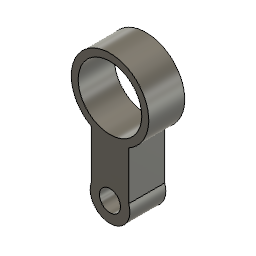
Trumpet+Clamp+4 (Autodesk Fusion 360 design; units mm, degrees)
Autodesk Fusion 360 part; units mm, degrees
note: some values were not read from the file. Chosen so that the rebuilt part matches the saved one: which face or edge a step refers to.
sketch "Sketch1" plane through (0, 0, 0) normal (0, 0, 1) x (1, 0, 0)
  circle A0 centre (0, 0) radius 2.25
  circle A1 centre (0, 0) radius 4.25
  line L0 (-4, 1.4361) -> (-4, 11.756)
  line L1 (4, 1.4361) -> (4, 11.756)
  circle A2 centre (0, 19) radius 6.775
  circle A3 centre (0, 19) radius 8.275
  line L2 (-4, 1.4361) -> (4, 1.4361) construction
  line L3 (-4, 11.756) -> (4, 11.756) construction
  line L4 (-2.7954, 26.7885) -> (-7.7596, 21.8747) construction
  line L5 (0, 0) -> (0, 19) construction
  dimension "d1" = 4.5
  dimension "d2" = 8.5
  dimension "d3" = 13.55
  dimension "d4" = 16.55
  dimension "d5" = 19
  dimension "d6" = 8
  constraint coincident A0.centre A1.centre
  constraint coincident A1 L0.start
  constraint coincident A1 L1.start
  constraint concentric A2 A3
  constraint parallel L0 L1
  constraint coincident L0.end A3
  constraint coincident L1.end A3
  constraint perpendicular L0 L2
  constraint perpendicular L0 L3
  constraint coincident A3 L4.end
  constraint coincident A3 L4.start
  constraint coincident A2.centre A3.centre
  constraint vertical L5
  measures "d1" diameter of A0
  measures "d2" diameter of A1
  measures "d3" diameter of A2
  measures "d4" diameter of A3
  measures "d5" distance of A0.centre A2.centre
  measures "d6" distance of L0 L1
extrude "Extrude1" add sketch "Sketch1" along normal blind 7.7
sketch "Sketch2" plane through (-2.8621, 2.7943, 0) normal (-0.715528, 0.698585, 0) x (0, 0, 1)
  line L0 (0, 10.5084) -> (0, 1.4361)
  line L1 (0, 1.4361) -> (7.7, 1.4361)
  line L2 (7.7, 1.4361) -> (7.7, 10.5084)
  line L3 (7.7, 10.5084) -> (0, 10.5084)
  line L4 (0, 5.9723) -> (7.7, 5.9723) construction
  line L5 (3.85, 10.5084) -> (3.85, 1.4361) construction
  circle A0 centre (3.85, 5.9723) radius 2.25
  dimension "d10" = 4.5
  constraint midpoint L0 L4.start
  constraint midpoint L2 L4.end
  constraint midpoint L3 L5.start
  constraint midpoint L1 L5.end
  constraint midpoint L5 A0.centre
  measures "d10" diameter of A0
extrude "Extrude2" [rolled back] side1offset 0 taper angle 0
sketch "Sketch3" plane through (15.0791, 0, 0) normal (1, 0, 0) x (0, 0, -1)
  line L0 (0, 19.0835) -> (0, 31.0835)
  line L1 (0, 31.0835) -> (-7.7, 31.0835)
  line L2 (-7.7, 31.0835) -> (-7.7, 19.0835)
  line L3 (-7.7, 19.0835) -> (0, 19.0835)
  line L4 (-3.85, 19.0835) -> (-3.85, 31.0835) construction
  line L5 (0, 25.0835) -> (-7.7, 25.0835) construction
  circle A0 centre (-3.85, 25.0835) radius 2.25
  dimension "d13" = 4.5
  constraint midpoint L3 L4.start
  constraint midpoint L1 L4.end
  constraint midpoint L0 L5.start
  constraint midpoint L2 L5.end
  constraint midpoint L4 A0.centre
  measures "d13" diameter of A0
extrude "Extrude3" [rolled back] side1offset 0 taper angle 0
equation "d4 = d3 + 3 mm"
